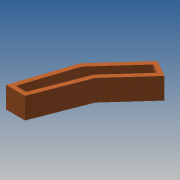
# Autodesk Inventor part: planter
Saved by Autodesk Inventor 2013 (Build 170138000, 138)
## iProperties
Created: 2014-01-02
Part Number: planter
Material: Wood (Cherry)
Document SubType Name: Modeling
Designer: ddeboer
Mass: 115971 g
Surface Area: 63041.1 cm^2
Volume: 231942 cm^3
Density: 0.5 g/cm^3
Author: ddeboer
Autodesk Inventor part; units mm, degrees
ref_plane "YZ Plane" through (0, 0, 0) normal (1, 0, 0) x (0, 1, 0)
ref_plane "XZ Plane" through (0, 0, 0) normal (0, 1, 0) x (-1, 0, 0)
ref_plane "XY Plane" through (0, 0, 0) normal (0, 0, 1) x (1, 0, 0)
sketch "Sketch1" plane through (0, 0, 0) normal (0, 1, 0) x (-1, 0, 0)
  line L0 (0, 0) -> (4480.984, 1200.676) construction
  line L1 (114.7485, 0) -> (3696.7474, 2068.068) construction
  line L2 (4480.984, 1200.676) -> (3696.7474, 2068.068) construction
  line L3 (0, 0) -> (4876.8, 0) construction
  line L4 (4480.984, 1200.676) -> (4876.8, 0) construction
  line L5 (4876.8, 0) -> (4470.4, 0)
  line L6 (3696.7474, 2068.068) -> (3344.7946, 1864.868) construction
  line L7 (3344.7946, 1864.868) -> (4049.7766, 1085.1344) construction
  line L8 (4049.7766, 1085.1344) -> (4470.4, 0) construction
  line L9 (0, 0) -> (4480.984, -1200.676) construction
  line L10 (114.7485, 0) -> (3696.7474, -2068.068) construction
  line L11 (4480.984, -1200.676) -> (3696.7474, -2068.068)
  line L12 (4480.984, -1200.676) -> (4876.8, 0)
  line L13 (3696.7474, -2068.068) -> (3344.7946, -1864.868)
  line L14 (3344.7946, -1864.868) -> (4049.7766, -1085.1344)
  line L15 (4049.7766, -1085.1344) -> (4470.4, 0)
  dimension "d3" = 4639.056
  dimension "d5" = 4136.136
  dimension "d7" = 4876.8
  dimension "d8" = 406.4
  dimension "d9" = 406.4
  constraints: 32 end point, 6 point on line, 4 symmetric about line, 1 parallel
  measures "d3" distance of L0.start L0.end
  measures "d5" distance of L1.start L1.end
  measures "d7" distance of L0.start L3.end
  measures "d8" distance of L3.end L5.end
  measures "d9" distance of L1.end L6.end
extrude "Extrusion1" add sketch "Sketch1" along normal blind 457.2
sketch "Sketch3" plane through (0, 457.2, 0) normal (0, 1, 0) x (1, 0, 0)
  line L0 (-4876.8, 0) -> (-4470.4, 0) projected
  line L1 (-4470.4, 0) -> (-4049.7766, 1085.1344) projected
  line L2 (-4049.7766, 1085.1344) -> (-3344.7946, 1864.868) projected
  line L3 (-3344.7946, 1864.868) -> (-3696.7474, 2068.068) projected
  line L4 (-3696.7474, 2068.068) -> (-4480.984, 1200.676) projected
  line L5 (-4480.984, 1200.676) -> (-4876.8, 0) projected
  line L6 (-4402.4373, 1154.9946) -> (-3678.9832, 1955.159)
  line L7 (-3678.9832, 1955.159) -> (-3484.5189, 1842.885)
  line L8 (-3484.5189, 1842.885) -> (-4126.7324, 1132.5754)
  line L9 (-4126.7324, 1132.5754) -> (-4531.2854, 88.9)
  line L10 (-4531.2854, 88.9) -> (-4753.887, 88.9)
  line L11 (-4753.887, 88.9) -> (-4402.4373, 1154.9946)
  point P0 (0, 0)
  dimension "d15" = 88.9
  constraints: 12 end point, 5 other
  measures "d15" distance between parallel lines of L6 L4
extrude "Extrusion3" cut sketch "Sketch3" against normal blind 406.4 contours L6 L7 L8 L9 L10 L11
body "Solid1"
